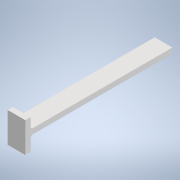
# Autodesk Inventor part: fence
Saved by Autodesk Inventor 2020 (Build 240168000, 168)
## iProperties
Created: 2019-05-08
Part Number: fence
Material: Generic
Document SubType Name: Modeling
Designer: erwin
Density: 1 g/cm^3
Appearance: Default
Author: erwin
Autodesk Inventor part; units mm, degrees
ref_plane "YZ Plane" through (0, 0, 0) normal (1, 0, 0) x (0, 1, 0)
ref_plane "XZ Plane" through (0, 0, 0) normal (0, 1, 0) x (-1, 0, 0)
ref_plane "XY Plane" through (0, 0, 0) normal (0, 0, 1) x (1, 0, 0)
sketch "Sketch1" plane through (0, 0, 0) normal (0, 0, 1) x (1, 0, 0)
  arc A0 (16, 5) -> (14, 7) centre (14, 5) ccw projected
  line L0 (14, 7) -> (8, 7) projected
  arc A1 (6, 9) -> (8, 7) centre (8, 9) ccw projected
  line L1 (6, 9) -> (6, 25.5) projected
  arc A2 (6, 25.5) -> (4, 27.5) centre (4, 25.5) ccw projected
  line L2 (4, 27.5) -> (-14, 27.5) projected
  arc A3 (-14, 27.5) -> (-16, 25.5) centre (-14, 25.5) ccw projected
  line L3 (-16, 25.5) -> (-16, 20.5) projected
  line L4 (-16, 20.5) -> (4, 20.5) projected
  line L5 (4, 20.5) -> (4, 5) projected
  line L6 (4, 5) -> (14, 5) projected
  line L7 (14, 5) -> (14, -15) projected
  line L8 (14, -15) -> (4, -15) projected
  line L9 (4, -15) -> (4, -20.5) projected
  line L10 (4, -20.5) -> (-16, -20.5) projected
  line L11 (-16, -20.5) -> (-16, -25.5) projected
  arc A4 (-16, -25.5) -> (-14, -27.5) centre (-14, -25.5) ccw projected
  line L12 (-14, -27.5) -> (4, -27.5) projected
  arc A5 (4, -27.5) -> (6, -25.5) centre (4, -25.5) ccw projected
  line L13 (6, -25.5) -> (6, -19) projected
  arc A6 (8, -17) -> (6, -19) centre (8, -19) ccw projected
  line L14 (8, -17) -> (14, -17) projected
  arc A7 (14, -17) -> (16, -15) centre (14, -15) ccw projected
  line L15 (16, -15) -> (16, 5) projected
  circle A8 centre (-10.2273, -23.9687) radius 0.75 projected
  circle A9 centre (-0.7, 24) radius 0.75 projected
  circle A10 centre (-10.2, 24) radius 0.75 projected
  circle A11 centre (-0.7, -24) radius 0.75 projected
  line L16 (14, 5) -> (4, 5)
  line L17 (4, 5) -> (4, 2)
  line L18 (4, 2) -> (14, 2)
  line L19 (14, 2) -> (14, 5)
  point P0 (0, 0)
  constraints: 8 end point, 2 parallel, 1 horizontal, 1 perpendicular, 1 other
extrude "Extrusion1" add sketch "Sketch1" along normal blind 80 contours L6 L7 L18 L17
sketch "Sketch2" plane through (0, 0, 80) normal (0, 0, 1) x (1, 0, 0)
  line L0 (14, 2) -> (14, 5) projected
  line L1 (14, 5) -> (4, 5) projected
  line L2 (4, 5) -> (4, 2) projected
  line L3 (4, 2) -> (14, 2) projected
  line L4 (14, 2) -> (4, 2)
  line L5 (4, 2) -> (4, -6)
  line L6 (4, -6) -> (14, -6)
  line L7 (14, -6) -> (14, 2)
  line L8 (14, 5) -> (4, 5)
  line L9 (4, 5) -> (4, 11)
  line L10 (4, 11) -> (14, 11)
  line L11 (14, 11) -> (14, 5)
  point P0 (0, 0)
  dimension "d2" = 8
  dimension "d3" = 6
  constraints: 16 end point, 4 parallel, 2 horizontal, 2 perpendicular
  measures "d2" distance of L5.end L4.end
  measures "d3" distance of L8.end L9.end
extrude "Extrusion2" add sketch "Sketch2" along normal blind 3
chamfer "Chamfer1" distance 1 angle 45 2 edges at (9, 2, 80) (9, 5, 80)
body "Solid1"
